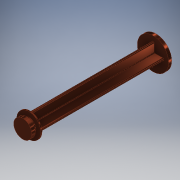
# Autodesk Inventor part: Plunger
Saved by Autodesk Inventor 2018 (Build 220112000, 112)
## iProperties
Created: 2019-11-16
Part Number: Plunger
Material: Generic
Document SubType Name: Modeling
Designer: ASUS
Density: 1 g/cm^3
Appearance: Copper - Polished
Author: ASUS
Autodesk Inventor part; units mm, degrees
ref_plane "YZ Plane" through (0, 0, 0) normal (1, 0, 0) x (0, 1, 0)
ref_plane "XZ Plane" through (0, 0, 0) normal (0, 1, 0) x (-1, 0, 0)
ref_plane "XY Plane" through (0, 0, 0) normal (0, 0, 1) x (1, 0, 0)
sketch "Sketch1" plane through (0, 0, 0) normal (0, 0, 1) x (1, 0, 0)
  line L0 (0, 5.5944) -> (0, -0.4056)
  line L1 (0, -0.4056) -> (7.5, -0.4056)
  line L2 (7.5, -0.4056) -> (7.5, 2.5944)
  line L3 (7.5, 2.5944) -> (6, 2.5944)
  line L4 (6, 2.5944) -> (6, 4.5944)
  line L5 (6, 4.5944) -> (10, 4.5944)
  line L6 (10, 4.5944) -> (10, 5.5944)
  line L7 (10, 5.5944) -> (0, 5.5944)
  point P0 (0, 0)
  dimension "d0" = 10
  dimension "d1" = 6
  dimension "d2" = 1
  dimension "d3" = 2
  dimension "d4" = 3
  dimension "d5" = 7.5
  constraints: 16 end point, 7 perpendicular, 1 vertical
  measures "d0" distance of L6.end L0.start
  measures "d1" distance between parallel lines of L4 L0
  measures "d2" distance of L5.end L6.end
  measures "d3" distance of L3.end L4.end
  measures "d4" distance of L1.end L2.end
  measures "d5" distance of L0.end L1.end
revolve "Revolution1" add sketch "Sketch1" angle 360 about axis through (0, 5.5944, 0) along (0, -1, 0)
sketch "Sketch2" plane through (0, 5.5944, 0) normal (0, 1, 0) x (1, 0, 0)
  arc A0 (1, 8) -> (-1, 8) centre (0, 8) ccw
  arc A1 (8, -1) -> (8, 1) centre (8, 0) ccw
  arc A2 (-1, -8) -> (1, -8) centre (0, -8) ccw
  arc A3 (-8, 1) -> (-8, -1) centre (-8, 0) ccw
  line L0 (-1, 8) -> (-1, 1.5)
  line L1 (-1, -1.5) -> (-1, -8)
  line L2 (1, 8) -> (1, 1.5)
  line L3 (1, -1.5) -> (1, -8)
  line L4 (-8, -1) -> (-1.5, -1)
  line L5 (1.5, -1) -> (8, -1)
  line L6 (-8, 1) -> (-1.5, 1)
  line L7 (1.5, 1) -> (8, 1)
  arc A4 (-1.5, 1) -> (-1, 1.5) centre (-1.5, 1.5) ccw
  arc A5 (1, 1.5) -> (1.5, 1) centre (1.5, 1.5) ccw
  arc A6 (-1, -1.5) -> (-1.5, -1) centre (-1.5, -1.5) ccw
  arc A7 (1.5, -1) -> (1, -1.5) centre (1.5, -1.5) ccw
  point P0 (0, 0)
  dimension "d11" = 8
  dimension "d16" = 8
  dimension "d17" = 8
  dimension "d18" = 8
  dimension "d19" = 0.5
  constraints: 16 end point, 16 point on circle, 16 tangent, 8 centre point, 4 horizontal, 4 vertical, 3 equal radius
  measures "d11" distance of point (0, 0) A0.centre
  measures "d16" distance of point (0, 0) A3.centre
  measures "d17" distance of A1.centre point (0, 0)
  measures "d18" distance of A2.centre point (0, 0)
  measures "d19" radius of A4
extrude "Extrusion1" add sketch "Sketch2" along normal blind 102
sketch "Sketch3" plane through (0, 107.5944, 0) normal (0, 1, 0) x (1, 0, 0)
  circle A0 centre (0, 0) radius 13
  dimension "d22" = 26
  constraints: 1 centre point, 1 coincident
  measures "d22" diameter of A0
extrude "Extrusion2" add sketch "Sketch3" along normal blind 2.5
sketch "Sketch4" plane through (0, 110.0944, 0) normal (0, 1, 0) x (1, 0, 0)
  line L0 (10, -1.5) -> (0, -1.5)
  line L1 (10, 1.5) -> (0, 1.5)
  arc A0 (10, -1.5) -> (10, 1.5) centre (10, 0) ccw
  line L2 (8, 2.7) -> (0, 2.7)
  line L3 (8, 5.7) -> (0, 5.7)
  arc A1 (8, 2.7) -> (8, 5.7) centre (8, 4.2) ccw
  line L4 (0, 6.9) -> (6, 6.9)
  line L5 (0, 9.9) -> (6, 9.9)
  arc A2 (6, 6.9) -> (6, 9.9) centre (6, 8.4) ccw
  line L6 (8, -2.7) -> (0, -2.7)
  line L7 (8, -5.7) -> (0, -5.7)
  arc A3 (8, -5.7) -> (8, -2.7) centre (8, -4.2) ccw
  line L8 (6, -6.9) -> (0, -6.9)
  line L9 (6, -9.9) -> (0, -9.9)
  arc A4 (6, -9.9) -> (6, -6.9) centre (6, -8.4) ccw
  line L10 (-10, -1.5) -> (0, -1.5)
  line L11 (-10, 1.5) -> (0, 1.5)
  arc A5 (-10, 1.5) -> (-10, -1.5) centre (-10, 0) ccw
  line L12 (-8, 2.7) -> (0, 2.7)
  line L13 (-8, 5.7) -> (0, 5.7)
  arc A6 (-8, 5.7) -> (-8, 2.7) centre (-8, 4.2) ccw
  line L14 (0, 6.9) -> (-6, 6.9)
  line L15 (0, 9.9) -> (-6, 9.9)
  arc A7 (-6, 9.9) -> (-6, 6.9) centre (-6, 8.4) ccw
  line L16 (-8, -2.7) -> (0, -2.7)
  line L17 (-8, -5.7) -> (0, -5.7)
  arc A8 (-8, -2.7) -> (-8, -5.7) centre (-8, -4.2) ccw
  line L18 (-6, -6.9) -> (0, -6.9)
  line L19 (-6, -9.9) -> (0, -9.9)
  arc A9 (-6, -6.9) -> (-6, -9.9) centre (-6, -8.4) ccw
  point P0 (0, 0)
  dimension "d25" = 1.5
  dimension "d26" = 1.5
  dimension "d27" = 10
  dimension "d28" = 10
  dimension "d29" = 1.2
  dimension "d30" = 3
  dimension "d31" = 8
  dimension "d32" = 8
  dimension "d33" = 1.2
  dimension "d34" = 6
  dimension "d35" = 6
  dimension "d36" = 3
  dimension "d37" = 1.2
  dimension "d38" = 8
  dimension "d39" = 8
  dimension "d40" = 3
  dimension "d41" = 1.2
  dimension "d42" = 3
  dimension "d43" = 6
  dimension "d44" = 6
  constraints: 40 end point, 20 point on circle, 10 centre point, 10 horizontal, 5 tangent
  measures "d25" distance from line of L0 point (0, 0)
  measures "d26" distance from line of L1 point (0, 0)
  measures "d27" distance of L0.start L0.end
  measures "d28" distance of L1.start L1.end
  measures "d29" distance between parallel lines of L2 L1
  measures "d30" distance between parallel lines of L3 L2
  measures "d31" distance of L2.start L2.end
  measures "d32" distance of L3.start L3.end
  measures "d33" distance between parallel lines of L3 L4
  measures "d34" distance of L5.start L5.end
  measures "d35" distance of L4.start L4.end
  measures "d36" distance between parallel lines of L5 L4
  measures "d37" distance between parallel lines of L6 L0
  measures "d38" distance of L7.start L7.end
  measures "d39" distance of L6.start L6.end
  measures "d40" distance between parallel lines of L7 L6
  measures "d41" distance between parallel lines of L8 L7
  measures "d42" distance between parallel lines of L9 L8
  measures "d43" distance of L8.start L8.end
  measures "d44" distance of L9.start L9.end
extrude "Extrusion3" add sketch "Sketch4" along normal blind 1
fillet "Fillet1" radius 1 20 edges at (7.5, 111.0944, -8.4) (0, 111.0944, -9.9) (-7.5, 111.0944, -8.4) (0, 111.0944, -6.9) (9.5, 111.0944, -4.2) (0, 111.0944, -5.7) (-9.5, 111.0944, -4.2) (0, 111.0944, -2.7) (11.5, 111.0944, 0) (0, 111.0944, -1.5) (-11.5, 111.0944, 0) (0, 111.0944, 1.5) (9.5, 111.0944, 4.2) (0, 111.0944, 2.7) (-9.5, 111.0944, 4.2) (0, 111.0944, 5.7) (7.5, 111.0944, 8.4) (0, 111.0944, 6.9) (-7.5, 111.0944, 8.4) (0, 111.0944, 9.9)
body "Solid1"
